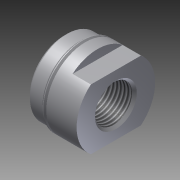
# Autodesk Inventor part: 040000_rear_head
Saved by Autodesk Inventor 2012 (Build 160160000, 160)
## iProperties
Category: PARTsolutions
Company: BIMBA
Created: 2013-01-17
Part Number: 040000_rear_head
Material: Default
Catalog Web Link: www.cadenas.de
Description: Rear Head-Original Line - Standard Air Cylinders
Vendor: BIMBA
Document SubType Name: Modeling
Designer: William
Manufacturer: BIMBA
Density: 1 g/cm^3
Mass: 3.07279 g
Surface Area: 18.9574 cm^2
Volume: 3.07279 cm^3
PSOL_IDENT_0: {\\10.0.0.242\data_v9\23d-libs\bimba\bimba\bimba_imperial\bimba_full_line\original_line_cylinders\st
PSOL_IDENT_1: andard_air_cylinders\rear_head.prj},227 {VTYP=3D},{NB=040000_rear_head},{LINA=040000_rear_head},{NN=
PSOL_IDENT_2: Rear Head},{DATE=24.09.2012 07:58:44},{GEOMDATE=24.09.2012 00:00:00},{VERSION=},{LINEID=40},{LINESUB
PSOL_IDENT_3: ID=-1},{WBVAR=MNT,ACTING,DER,Q,T1,T2,T3,T4,TRIM,Y,K,MB,CUSH,FBON}  {NB=040000_rear_head},{LINA=04000
PSOL_IDENT_4: 0_rear_head},{KT=DUMMY},{PN=040000},{BORE=0.75000},{BOREPN=04},{MNT=},{MNTALG='' , 'Front Nose' , 'P
PSOL_IDENT_5: ' , 'Rear Pivot' , 'LS' , 'Built-in Valve LS' , 'DX' , 'Double End' , 'BR' , 'Rear Block' , 'BRT' ,
PSOL_IDENT_6: 'Rear Trunnion' , 'A' , 'Adjustable Stroke'},{ACTING=},{ACTINGALG= '' , 'Single Acting' , 'R' , 'Rev
PSOL_IDENT_7: erse/Double Acting'   },{DER=},{DERALG= '' , 'Standard' },{Q=},{T1=},{T2=},{T3=},{T4=},{TRIM=0},{Y=}
PSOL_IDENT_8: ,{K=},{KALG= '', 'without K', 'K', 'with K' },{MB=0},{A1=0.5310},{A1N=0.5310},{A1P=1.5940},{A1B=1.09
PSOL_IDENT_9: 40},{A1S=1.2190},{A2=0.219},{A2N=0.2190},{A3=0.0300},{D1=0.8050},{D1N=0.8050},{D1P=0.8625},{D1B=0.83
PSOL_IDENT_10: 25},{D2=0.7615},{C1=0.0300},{C2=0.0000},{NDM=0.4050},{TAB=NPT},{NDMDP=0.3020},{D3=0.3440},{A4=0.1880
PSOL_IDENT_11: },{A5=0.6200},{D4=0.0000},{A6=0.0000},{A7=0.7500},{A8=0.1250},{D5=0.8170},{D6=0.3120},{A9=0.8440},{N
PSOL_IDENT_12: DM2=0.6250},{TAB2=UNF},{C11=0.0300},{C22=0.0000},{C33=0.0227},{C44=0.0300},{A10=0.3725},{A11=0.0000}
PSOL_IDENT_13: ,{NDM3=0.4050},{NDM3N=0.4050},{NDM3B=0.4050},{TAB3=NPT},{TAB3N=NPT},{TAB3B=NPT},{A12=0.688},{A12N=0.
PSOL_IDENT_14: 6880},{A12B=0.6560},{A13=1.3120},{D7=0.2520},{D8=0.6225},{A14=0.0940},{A15=0.0855},{D9=0.5385},{R1=0
PSOL_IDENT_15: .0350},{X1=0.0000},{X2=0.0000},{CX=0.0000},{CC=0.0000},{CON=0},{S1=1.0000},{DB=0.2500},{X1B=0.4380},
PSOL_IDENT_16: {X2B=0.0310},{A8B=0.1250},{A9B=0.8750},{MODEL=1},{NDM4=0.1900},{TAB4=UNF},{NDM4DP=0.2500},{BC=1.0000
PSOL_IDENT_17: },{B1=0.7150},{B2=0.5000},{B3=0.5000},{ON=0},{ON2=1},{G1=0.1250},{G2=0.5620},{G3=0.6250},{G4=0.6250}
PSOL_IDENT_18: ,{GD=0.2520},{G5=0.6250},{G6=0.3725},{RON=0},{H1=1.1175},{H2=0.8170},{H3=0.1250},{H4=0.0350},{H5=0.9
PSOL_IDENT_19: 420},{H6=0.5620},{F=0.4380},{PNUT=0.0000},{CUSH=0},{CC11=0.238},{CC111=0.2380},{CC22=0.2750},{CC33=0
PSOL_IDENT_20: .1950},{CC44=0.3700},{CC55=0.5350},{CD1=0.1900},{CD2=0.1500},{CD3=0.0725},{CNDM3=0.1380},{CTAB3=UNF}
PSOL_IDENT_21: ,{OLEN=0.5310},{OD=0.3455},{STDIS=0.1560},{STDIS1=0.1560},{BUSHCON=D-3543},{BUSHL=0.3700},{FBON=0},{
PSOL_IDENT_22: LCD=0.0000}
CNS_NT: Original Line - Standard Air Cylinders
CNS_NB: 040000_rear_head
CNS_NBSYN: $PN._rear_head
CNS_LINA: 040000_rear_head
CNS_PN: 040000
CNS_BORE: 0.75000
CNS_BOREPN: 04
CNS_MNT: Front Nose
CNS_MNTALG: '' , 'Front Nose' , 'P' , 'Rear Pivot' , 'LS' , 'Built-in Valve LS' , 'DX' , 'Double End' , 'BR' , 'Rear Block' , 'BRT' , 'Rear Trunnion' , 'A' , 'Adjustable Stroke'
CNS_ACTING: Single Acting
CNS_ACTINGALG: '' , 'Single Acting' , 'R' , 'Reverse/Double Acting'
CNS_DER: Standard
CNS_DERALG: '' , 'Standard'
CNS_Q: Without Side Ported Rear Head
CNS_T1: without T1
CNS_T2: without T2
CNS_T3: without T3
CNS_T4: without T4
CNS_TRIM: 0
CNS_Y: without Pivot Bushing
CNS_K: without K
CNS_KALG: '', 'without K', 'K', 'with K'
CNS_MB: 0
CNS_A1: 0.5310
CNS_A1N: 0.5310
CNS_A1P: 1.5940
CNS_A1B: 1.0940
CNS_A1S: 1.2190
CNS_A2: 0.219
CNS_A2N: 0.2190
CNS_A3: 0.0300
CNS_D1: 0.8050
CNS_D1N: 0.8050
CNS_D1P: 0.8625
CNS_D1B: 0.8325
CNS_D2: 0.7615
CNS_C1: 0.0300
CNS_C2: 0.0000
CNS_NDM: 0.4050
CNS_TAB: NPT
CNS_NDMDP: 0.3020
CNS_D3: 0.3440
CNS_A4: 0.1880
CNS_A5: 0.6200
CNS_D4: 0.0000
CNS_A6: 0.0000
CNS_A7: 0.7500
CNS_A8: 0.1250
CNS_D5: 0.8170
CNS_D6: 0.3120
CNS_A9: 0.8440
CNS_NDM2: 0.6250
CNS_TAB2: UNF
CNS_C11: 0.0300
CNS_C22: 0.0000
CNS_C33: 0.0227
CNS_C44: 0.0300
CNS_A10: 0.3725
CNS_A11: 0.0000
CNS_NDM3: 0.4050
CNS_NDM3N: 0.4050
CNS_NDM3B: 0.4050
CNS_TAB3: NPT
CNS_TAB3N: NPT
CNS_TAB3B: NPT
CNS_A12: 0.688
CNS_A12N: 0.6880
CNS_A12B: 0.6560
CNS_A13: 1.3120
CNS_D7: 0.2520
CNS_D8: 0.6225
CNS_A14: 0.0940
CNS_A15: 0.0855
CNS_D9: 0.5385
CNS_R1: 0.0350
CNS_X1: 0.0000
CNS_X2: 0.0000
CNS_CX: 0.0000
CNS_CC: 0.0000
CNS_CON: 0
CNS_S1: 1.0000
CNS_DB: 0.2500
CNS_X1B: 0.4380
CNS_X2B: 0.0310
CNS_A8B: 0.1250
CNS_A9B: 0.8750
CNS_MODEL: 1
CNS_NDM4: 0.1900
CNS_TAB4: UNF
CNS_NDM4DP: 0.2500
CNS_BC: 1.0000
CNS_B1: 0.7150
CNS_B2: 0.5000
CNS_B3: 0.5000
CNS_ON: 0
CNS_ON2: 1
CNS_G1: 0.1250
CNS_G2: 0.5620
CNS_G3: 0.6250
CNS_G4: 0.6250
CNS_GD: 0.2520
CNS_G5: 0.6250
CNS_G6: 0.3725
CNS_RON: 0
CNS_H1: 1.1175
CNS_H2: 0.8170
CNS_H3: 0.1250
CNS_H4: 0.0350
CNS_H5: 0.9420
CNS_H6: 0.5620
CNS_F: 0.4380
CNS_PNUT: 0.0000
CNS_CUSH: 0
CNS_CC11: 0.238
CNS_CC111: 0.2380
CNS_CC22: 0.2750
CNS_CC33: 0.1950
CNS_CC44: 0.3700
CNS_CC55: 0.5350
CNS_CD1: 0.1900
CNS_CD2: 0.1500
CNS_CD3: 0.0725
CNS_CNDM3: 0.1380
CNS_CTAB3: UNF
CNS_OLEN: 0.5310
CNS_OD: 0.3455
CNS_STDIS: 0.1560
CNS_STDIS1: 0.1560
CNS_BUSHCON: D-3543
CNS_BUSHL: 0.3700
CNS_FBON: 0
CNS_LCD: 0.0000
SUPPLIER: BIMBA
ARTICLENO: 040000_rear_head
BOMINFO: 040000_rear_head
CREATOR: CADENAS GmbH
Title: 040000_rear_head
Author: Cadenas PARTsolutions
Comments: Original Line - Standard Air Cylinders
Autodesk Inventor part; units mm, degrees
sketch "Sketch_1" plane through (0, 0, 0) normal (0, 0, 1) x (1, 0, 0)
  line L0 (13.4874, 0) -> (0, 0)
  line L1 (0, 0) -> (0, 8.9091)
  line L2 (0, 8.9091) -> (0.762, 9.671)
  line L3 (0.762, 9.671) -> (4.0386, 9.671)
  line L4 (4.0386, 9.671) -> (4.8006, 8.9091)
  line L5 (4.8006, 8.9091) -> (5.5626, 8.9091)
  line L6 (5.5626, 8.9091) -> (5.5626, 10.2235)
  line L7 (5.5626, 10.2235) -> (13.4874, 10.2235)
  line L8 (13.4874, 10.2235) -> (13.4874, 0)
  line L9 (13.4874, 0) -> (0, 0)
  constraints: 20 end point
revolve "Revolution1" add sketch "Sketch_1" angle 360 about axis through (13.4874, 0, 0) along (1, 0, 0)
sketch "Sketch_6" plane through (0, 0, 0) normal (0, 0, 1) x (1, 0, 0)
  line L0 (13.4874, 0) -> (0, 0)
  line L1 (0, 0) -> (0, 4.3688)
  line L2 (0, 4.3688) -> (-1.5889, 4.3688)
  line L3 (-1.5889, 4.3688) -> (12.8524, 4.8197)
  line L4 (12.8524, 4.8197) -> (13.4874, 5.4547)
  line L5 (13.4874, 5.4547) -> (13.4874, 0)
  line L6 (13.4874, 0) -> (0, 0)
  constraints: 14 end point
revolve "Revolution2" cut sketch "Sketch_6" angle 360 about axis through (13.4874, 0, 0) along (1, 0, 0)
thread "Thread1" size "1/8" designation "1/8 - 27 NPT" standard "NPT" length 7.6708 offset 5.8029
sketch "Sketch_5" plane through (13.4874, 0, 0) normal (1, 0, 0) x (0, 0, -1)
  line L0 (-40.894, 20.447) -> (-40.894, -20.447)
  line L1 (-40.894, -20.447) -> (40.894, -20.447)
  line L2 (40.894, -20.447) -> (40.894, 20.447)
  line L3 (40.894, 20.447) -> (-40.894, 20.447)
  line L4 (-20.447, 7.874) -> (-20.447, -7.874)
  line L5 (-20.447, -7.874) -> (20.447, -7.874)
  line L6 (20.447, -7.874) -> (20.447, 7.874)
  line L7 (20.447, 7.874) -> (-20.447, 7.874)
  constraints: 16 end point
extrude "Extrusion1" cut sketch "Sketch_5" against normal blind 4.7752
sketch "Sketch_24" plane through (0, 0, 0) normal (0, 0, 1) x (1, 0, 0)
  line L0 (5.5626, 0) -> (4.8006, 0)
  line L1 (4.6479, 10.1393) -> (5.4401, 9.3472)
  arc A0 (5.4401, 9.1676) -> (5.4401, 9.3472) centre (5.3503, 9.2574) ccw
  line L2 (5.4401, 9.1676) -> (5.1816, 8.9091)
  line L3 (5.1816, 8.9091) -> (4.8006, 8.9091)
  line L4 (4.8006, 8.9091) -> (4.8006, 8.655)
  line L5 (4.8006, 8.655) -> (5.5626, 8.655)
  line L6 (5.5626, 8.655) -> (5.5626, 9.512)
  line L7 (5.5626, 9.512) -> (4.8511, 10.2235)
  line L8 (4.8511, 10.2235) -> (4.6479, 10.2235)
  line L9 (4.6479, 10.2235) -> (4.6479, 10.1393)
  constraints: 20 end point, 2 point on circle, 1 centre point
revolve "Revolution3" add sketch "Sketch_24" angle 360 about axis through (5.5626, 0, 0) along (1, 0, 0)
ref_plane "cut1_XY" through (13.4874, 7.874, 0) normal (1, 0, 0) x (0, 0, -1)
ref_plane "cut1_YZ" through (13.4874, 7.874, 0) normal (0, 0, -1) x (0, 1, 0)
ref_plane "cut1_ZX" through (13.4874, 7.874, 0) normal (0, 1, 0) x (1, 0, 0)
ref_plane "cut2_XY" through (13.4874, -7.874, 0) normal (1, 0, 0) x (0, 0, -1)
ref_plane "cut2_YZ" through (13.4874, -7.874, 0) normal (0, 0, -1) x (0, 1, 0)
ref_plane "cut2_ZX" through (13.4874, -7.874, 0) normal (0, 1, 0) x (1, 0, 0)
ref_plane "to_tube_XY" through (4.8006, 0, 0) normal (1, 0, 0) x (0, 0, -1)
ref_plane "to_tube_YZ" through (4.8006, 0, 0) normal (0, 0, -1) x (0, 1, 0)
ref_plane "to_tube_ZX" through (4.8006, 0, 0) normal (0, 1, 0) x (1, 0, 0)
ref_plane "lovra_XY" through (13.4874, 0, 0) normal (1, 0, 0) x (0, 1, 0)
ref_plane "lovra_YZ" through (13.4874, 0, 0) normal (0, 1, 0) x (0, 0, 1)
ref_plane "lovra_ZX" through (13.4874, 0, 0) normal (0, 0, 1) x (1, 0, 0)
ref_plane "to_nut_XY" through (0, 0, 0) normal (1, 0, 0) x (0, 0, -1)
ref_plane "to_nut_YZ" through (0, 0, 0) normal (0, 0, -1) x (0, 1, 0)
ref_plane "to_nut_ZX" through (0, 0, 0) normal (0, 1, 0) x (1, 0, 0)
ref_plane "lovra1_XY" through (8.7122, 0, 0) normal (1, 0, 0) x (0, 0, -1)
ref_plane "lovra1_YZ" through (8.7122, 0, 0) normal (0, 0, -1) x (0, 1, 0)
ref_plane "lovra1_ZX" through (8.7122, 0, 0) normal (0, 1, 0) x (1, 0, 0)
ref_plane "lovra2_XY" through (8.7122, 7.874, 0) normal (1, 0, 0) x (0, 0, -1)
ref_plane "lovra2_YZ" through (8.7122, 7.874, 0) normal (0, 0, -1) x (0, 1, 0)
ref_plane "lovra2_ZX" through (8.7122, 7.874, 0) normal (0, 1, 0) x (1, 0, 0)
ref_plane "lovra3_XY" through (8.7122, -7.874, 0) normal (1, 0, 0) x (0, 0, -1)
ref_plane "lovra3_YZ" through (8.7122, -7.874, 0) normal (0, 0, -1) x (0, 1, 0)
ref_plane "lovra3_ZX" through (8.7122, -7.874, 0) normal (0, 1, 0) x (1, 0, 0)
ref_plane "to_pin_XY" through (33.3248, 0, 0) normal (0, 0, 1) x (1, 0, 0)
ref_plane "to_pin_YZ" through (33.3248, 0, 0) normal (1, 0, 0) x (0, 1, 0)
ref_plane "to_pin_ZX" through (33.3248, 0, 0) normal (0, 1, 0) x (0, 0, 1)
ref_plane "olen_XY" through (13.4874, 0, 0) normal (1, 0, 0) x (0, 0, -1)
ref_plane "olen_YZ" through (13.4874, 0, 0) normal (0, 0, -1) x (0, 1, 0)
ref_plane "olen_ZX" through (13.4874, 0, 0) normal (0, 1, 0) x (1, 0, 0)
ref_plane "cutf1_XY" through (13.4874, 0, 0) normal (0, 0, 1) x (1, 0, 0)
ref_plane "cutf1_YZ" through (13.4874, 0, 0) normal (1, 0, 0) x (0, 1, 0)
ref_plane "cutf1_ZX" through (13.4874, 0, 0) normal (0, 1, 0) x (0, 0, 1)
ref_plane "cutf2_XY" through (8.7122, 0, 0) normal (0, 0, 1) x (1, 0, 0)
ref_plane "cutf2_YZ" through (8.7122, 0, 0) normal (1, 0, 0) x (0, 1, 0)
ref_plane "cutf2_ZX" through (8.7122, 0, 0) normal (0, 1, 0) x (0, 0, 1)
ref_plane "lovra21_XY" through (0, 0, 5.2705) normal (1, 0, 0) x (0, 0, -1)
ref_plane "lovra21_YZ" through (0, 0, 5.2705) normal (0, 0, -1) x (0, 1, 0)
ref_plane "lovra21_ZX" through (0, 0, 5.2705) normal (0, 1, 0) x (1, 0, 0)
ref_plane "lovra22_XY" through (0, 0, -5.2705) normal (1, 0, 0) x (0, 0, -1)
ref_plane "lovra22_YZ" through (0, 0, -5.2705) normal (0, 0, -1) x (0, 1, 0)
ref_plane "lovra22_ZX" through (0, 0, -5.2705) normal (0, 1, 0) x (1, 0, 0)
ref_plane "to_screw_XY" through (17.4752, 2.032, -6.0452) normal (0, 1, 0) x (1, 0, 0)
ref_plane "to_screw_YZ" through (17.4752, 2.032, -6.0452) normal (1, 0, 0) x (0, 0, -1)
ref_plane "to_screw_ZX" through (17.4752, 2.032, -6.0452) normal (0, 0, -1) x (0, 1, 0)
ref_plane "to_mounting_bracket_XY" through (24.6126, 0, 0) normal (1, 0, 0) x (0, 0, -1)
ref_plane "to_mounting_bracket_YZ" through (24.6126, 0, 0) normal (0, 0, -1) x (0, 1, 0)
ref_plane "to_mounting_bracket_ZX" through (24.6126, 0, 0) normal (0, 1, 0) x (1, 0, 0)
body "Solid1"
